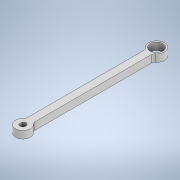
# Autodesk Inventor part: eslabon2
Saved by Autodesk Inventor 2021 (Build 250183000, 183)
## iProperties
Created: 2022-10-24
Part Number: eslabon2
Material: Genérico
Document SubType Name: Modeling
Designer: ivanm
Density: 1 g/cm^3
Appearance: Valor por defecto
Author: ivanm
Autodesk Inventor part; units mm, degrees
ref_plane "YZ Plane" through (0, 0, 0) normal (1, 0, 0) x (0, 1, 0)
ref_plane "XZ Plane" through (0, 0, 0) normal (0, 1, 0) x (-1, 0, 0)
ref_plane "XY Plane" through (0, 0, 0) normal (0, 0, 1) x (1, 0, 0)
sketch "Boceto2" plane through (0, 0, 0) normal (0, 1, 0) x (-1, 0, 0)
  arc A0 (5, 0) -> (-5, 0) centre (0, 0) ccw
  arc A1 (1.2, 2.1932) -> (1.2, -2.1932) centre (0, 0) ccw
  line L0 (1.2, 2.1932) -> (1.2, -2.1932)
  line L1 (0, 0) -> (0, -180) construction
  circle A2 centre (0, -180) radius 8.75
  arc A3 (-6.8254, -171.6948) -> (6.8254, -171.6948) centre (0, -180) ccw
  line L2 (5, -11.1803) -> (5, -167.8319)
  line L3 (-5, -11.1803) -> (-5, -167.8319)
  arc A4 (-6.8254, -171.6948) -> (-5, -167.8319) centre (-10, -167.8319) ccw
  arc A5 (5, -167.8319) -> (6.8254, -171.6948) centre (10, -167.8319) ccw
  arc A6 (6.6667, -7.4536) -> (-6.6667, -7.4536) centre (0, 0) ccw
  arc A7 (6.6667, -7.4536) -> (5, -11.1803) centre (10, -11.1803) ccw
  arc A8 (-5, -11.1803) -> (-6.6667, -7.4536) centre (-10, -11.1803) ccw
  point P0 (-5, -170.4836)
  point P1 (5, -170.4836)
  point P2 (5, -8.6603)
  point P3 (-5, -8.6603)
  dimension "d13" = 10
  dimension "d14" = 5
  dimension "d15" = 1.2
  dimension "d16" = 180
  dimension "d17" = 17.5
  dimension "d18" = 2
  dimension "d19" = 5
  dimension "d27" = 20
  dimension "d28" = 5
  dimension "d29" = 5
  constraints: 20 point on circle, 10 tangent, 9 centre point, 8 end point, 5 coincident, 4 point on line, 3 vertical, 1 equal radius, 1 parallel
  measures "d13" diameter of A0
  measures "d14" diameter of A1
  measures "d15" distance from line of point (0, 0) L0
  measures "d16" distance of L1.start L1.end
  measures "d17" diameter of A2
  measures "d18" radial gap between concentric circles of A3 A2
  measures "d19" radius of A4
  measures "d27" diameter of A6
  measures "d28" radius of A7
  measures "d29" radius of A8
extrude "Extrusión2" add sketch "Boceto2" along normal blind 10
sketch "Boceto3" plane through (0, 10, 0) normal (0, 1, 0) x (1, 0, 0)
  circle A0 centre (0, 0) radius 4
  line L0 (-3, -2.6458) -> (-3, 2.6458)
  line L1 (-3, -2.6458) -> (4.3142, -2.6458) construction
  dimension "d22" = 8
  dimension "d25" = 90
  dimension "d26" = 3
  constraints: 4 end point, 2 point on circle, 1 centre point, 1 coincident, 1 horizontal
  measures "d22" diameter of A0
  measures "d25" angle of L1 L0
  measures "d26" distance from line of point (0, 0) L0
extrude "Extrusión3" cut sketch "Boceto3" against normal blind 10 contours A0 L0 picked at (0.3596, 0.8073)
